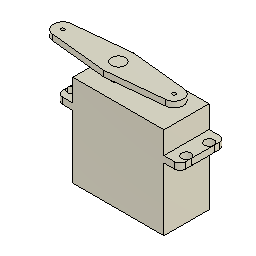
Trunk v2 (Autodesk Fusion 360 archive; units mm, degrees)
design "Servo"
Autodesk Fusion 360 part; units mm, degrees
sketch "Sketch1" plane through (0, 0, 0) normal (0, 1, 0) x (1, 0, 0)
  line L0 (0, 0) -> (39.6, 0)
  line L1 (39.6, 0) -> (39.6, -19.6)
  line L2 (39.6, -19.6) -> (0, -19.6)
  line L3 (0, -19.6) -> (0, 0)
  dimension "d1" = 19.6
  dimension "d2" = 39.6
  constraint horizontal L0
  constraint vertical L1
  constraint horizontal L2
  constraint vertical L3
  constraint coincident L0.start L3.end
  measures "d1" distance of L0.start L2.end
  measures "d2" distance of L1.end L2.end
extrude "Extrude1" add sketch "Sketch1" along normal blind 39.9 makes body 1
ref_plane "WorkPlane1" through (19.8, 27.4, 9.8) normal (0, -1, 0) x (-1, 0, 0)
sketch "Sketch2" plane through (0, 27.4, 0) normal (0, -1, 0) x (-1, 0, 0)
  line L0 (-46.6, -19.6) -> (7, -19.6)
  line L1 (7, -19.6) -> (7, 0)
  line L2 (7, 0) -> (-46.6, 0)
  line L3 (-46.6, 0) -> (-46.6, -19.6)
  line L4 (-46.6, -19.6) -> (7, 0) construction
  line L5 (7, -19.6) -> (-46.6, 0) construction
  line L6 (-19.8, -19.6) -> (-19.8, 0) construction
  line L7 (-39.6, -19.6) -> (0, -19.6) construction
  line L8 (0, 0) -> (-39.6, 0) construction
  circle A0 centre (-44.55, -14.8) radius 2.05
  circle A1 centre (-44.55, -4.8) radius 2.05
  circle A2 centre (4.95, -14.8) radius 2.05
  circle A3 centre (4.95, -4.8) radius 2.05
  line L9 (-44.55, -14.8) -> (4.95, -14.8) construction
  line L10 (4.95, -14.8) -> (4.95, -4.8) construction
  line L11 (4.95, -4.8) -> (-44.55, -4.8) construction
  line L12 (-44.55, -4.8) -> (-44.55, -14.8) construction
  line L13 (7, -9.8) -> (4.95, -9.8) construction
  point P0 (-19.8, -9.8)
  point P1 (-19.8, -14.8)
  dimension "d7" = 53.6
  dimension "d8" = 4.1
  dimension "d9" = 49.5
  dimension "d10" = 10
  constraint horizontal L0
  constraint perpendicular L0 L1
  constraint parallel L0 L2
  constraint parallel L1 L3
  constraint coincident L4 P0
  constraint coincident L5 P0
  constraint vertical L6
  constraint midpoint L6.start L7
  constraint midpoint L6.end L8
  constraint midpoint P0 L6
  constraint collinear L0 L7
  constraint horizontal L9
  constraint vertical L10
  constraint horizontal L11
  constraint vertical L12
  constraint coincident A3.centre L10.end
  constraint coincident A0.centre L9.start
  constraint coincident A1.centre L11.end
  constraint coincident A2.centre L9.end
  constraint equal A0 A1
  constraint equal A1 A3
  constraint equal A2 A3
  constraint coincident L6 P1
  constraint midpoint L9 P1
  constraint midpoint L1 L13.start
  constraint midpoint L10 L13.end
  constraint horizontal L13
  measures "d7" distance of L1 L3
  measures "d8" diameter of A0
  measures "d9" distance of A0.centre A2.centre
  measures "d10" distance of A0.centre A1.centre
extrude "Extrude2" add sketch "Sketch2" against normal blind 2.8 bodies 1
sketch "Sketch3" plane through (0, 39.9, 0) normal (0, 1, 0) x (-1, 0, 0)
  line L0 (0, 19.6) -> (-39.6, 19.6)
  line L1 (-39.6, 19.6) -> (-39.6, 0)
  line L2 (-39.6, 0) -> (0, 0)
  line L3 (0, 0) -> (0, 19.6)
  line L4 (0, 9.8) -> (-10, 9.8) construction
  circle A0 centre (-10, 9.8) radius 3
  dimension "d13" = 6
  dimension "d14" = 10
  constraint midpoint L3 L4.start
  constraint perpendicular L3 L4
  constraint coincident L4.end A0.centre
  measures "d13" diameter of A0
  measures "d14" distance of L4.start L4.end
extrude "Extrude3" add sketch "Sketch3" along normal blind 6 contours A0 bodies 1
fillet "Fillet1" radius 2.5 4 edges at (-7, 28.8, 19.6) (-7, 28.8, 0) (46.6, 28.8, 19.6) (46.6, 28.8, 0) on bodies 1
sketch "Sketch5" plane through (0, 45.9, 0) normal (0, 1, 0) x (-1, 0, 0)
  circle A0 centre (-10, 9.8) radius 3
  line L0 (6.25, 9.8) -> (-10, -6.45) construction
  line L1 (-10, -6.45) -> (-26.25, 9.8) construction
  line L2 (-26.25, 9.8) -> (-10, 26.05) construction
  line L3 (-10, 26.05) -> (6.25, 9.8) construction
  line L4 (-18.125, 17.925) -> (-1.875, 1.675) construction
  line L5 (-1.875, 17.925) -> (-18.125, 1.675) construction
  line L6 (-10, 9.8) -> (-7, 9.8) construction
  circle A1 centre (6.25, 9.8) radius 0.75
  circle A2 centre (-26.25, 9.8) radius 0.75
  circle A3 centre (-10, -6.45) radius 0.75
  circle A4 centre (-10, 26.05) radius 0.75
  line L7 (6.25, 13.8) -> (-26.25, 13.8)
  arc A5 (-26.25, 13.8) -> (-26.25, 5.8) centre (-26.25, 9.8) ccw
  line L8 (-26.25, 5.8) -> (6.25, 5.8)
  arc A6 (6.25, 5.8) -> (6.25, 13.8) centre (6.25, 9.8) ccw
  line L9 (6.25, 9.8) -> (-26.25, 9.8) construction
  line L10 (-6, -6.45) -> (-6, 26.05)
  arc A7 (-6, 26.05) -> (-14, 26.05) centre (-10, 26.05) ccw
  line L11 (-14, 26.05) -> (-14, -6.45)
  arc A8 (-14, -6.45) -> (-6, -6.45) centre (-10, -6.45) ccw
  line L12 (-10, -6.45) -> (-10, 26.05) construction
  point P0 (-10, 9.8)
  dimension "d34" = 45
  dimension "d35" = 32.5
  dimension "d36" = 1.5
  dimension "d37" = 4
  constraint perpendicular L0 L1
  constraint parallel L0 L2
  constraint parallel L1 L3
  constraint midpoint L2 L4.start
  constraint midpoint L0 L4.end
  constraint perpendicular L0 L4
  constraint midpoint L3 L5.start
  constraint midpoint L1 L5.end
  constraint coincident L4 P0
  constraint midpoint L5 P0
  constraint equal L4 L5
  constraint coincident P0 A0.centre
  constraint coincident A0 L6.end
  constraint horizontal L6
  constraint coincident L0.start L3.end
  constraint coincident L1.end L2.start
  constraint coincident L0.end L1.start
  constraint coincident L2.end L3.start
  constraint equal A2 A3
  constraint equal A1 A3
  constraint equal A1 A4
  constraint tangent L7 A5
  constraint tangent A5 L8
  constraint parallel L7 L8
  constraint tangent L8 A6
  constraint tangent L7 A6
  constraint horizontal L9
  constraint tangent L10 A7
  constraint tangent A7 L11
  constraint parallel L10 L11
  constraint tangent L11 A8
  constraint tangent L10 A8
  constraint vertical L12
  constraint equal A5 A8
  measures "d34" angle of L4 L6
  measures "d35" distance of L0.start L1.end
  measures "d36" diameter of A2
  measures "d37" radius of A8
extrude "Extrude6" add sketch "Sketch5" against normal blind 2.5 separate body makes body 2
copy_body "Body->Comp1" bodies 2 removing the originals makes body 3 in component "4 arm "
copy_body "Body->Comp2" bodies 1 removing the originals makes body 4 in component "Servo"
sketch "Sketch6" plane through (0, 45.9, 0) normal (0, 1, 0) x (-1, 0, 0)
  circle A0 centre (-10, 9.8) radius 3
  arc A1 (14.6568, 5.8207) -> (14.6568, 13.7793) centre (14.25, 9.8) ccw
  arc A2 (-34.6568, 13.7793) -> (-34.6568, 5.8207) centre (-34.25, 9.8) ccw
  line L0 (-34.25, 9.8) -> (14.25, 9.8) construction
  circle A3 centre (14.25, 9.8) radius 0.75
  circle A4 centre (-34.25, 9.8) radius 0.75
  line L1 (14.6568, 5.8207) -> (-10, 3.3)
  line L2 (-10, 3.3) -> (-34.6568, 5.8207)
  line L3 (-34.6568, 13.7793) -> (-10, 16.3)
  line L4 (-10, 16.3) -> (14.6568, 13.7793)
  line L5 (-10, 3.3) -> (-10, 16.3) construction
  circle A5 centre (-10, 9.8) radius 3
  point P0 (-10, 9.8)
  dimension "d46" = 48.5
  dimension "d48" = 1.5
  dimension "d49" = 13
  dimension "d50" = 4
  dimension "d51" = 6
  constraint horizontal L0
  constraint coincident P0 A0.centre
  constraint midpoint L0 P0
  constraint concentric A1 A3
  constraint concentric A2 A4
  constraint equal A3 A4
  constraint equal A1 A2
  constraint vertical L5
  constraint equal L1 L2
  constraint equal L3 L4
  constraint tangent A1 L1
  constraint tangent A1 L4
  constraint tangent A2 L3
  constraint midpoint P0 L5
  constraint concentric A0 A5
  measures "d46" distance of A2.centre A1.centre
  measures "d48" diameter of A3
  measures "d49" distance of L1.end L3.end
  measures "d50" radius of A1
  measures "d51" diameter of A5
extrude "Extrude7" add sketch "Sketch6" against normal blind 2.5 separate body makes body 5
copy_body "Body->Comp3" bodies 5 removing the originals makes body 6 in component "2 arm "
move_body "Move1" bodies 4 to x (1, 0, 0) y (0, 0, 1) z (0, -1, 0) at (0, 49.7, -30.1) in component "Servo"
move_body "Move1'" bodies 6 to x (1, 0, 0) y (0, 0, 1) z (0, -1, 0) at (0, 49.7, -30.1) in component "2 arm "
move_body "Move2" bodies 4 to x (1, 0, 0) y (0, 1, 0) z (0, 0, 1) at (0, -49.7, 30.1) in component "Servo"
move_body "Move2'" bodies 6 to x (1, 0, 0) y (0, 1, 0) z (0, 0, 1) at (0, -49.7, 30.1) in component "2 arm "
component "4 arm " placed x (1, 0, 0) y (0, 0, -1) z (0, 1, 0) at (0, -19.6, 89.3)
component "Servo" placed x (1, 0, 0) y (0, 1, 0) z (0, 0, 1) at (0, 0, 0)
component "2 arm " placed x (1, 0, 0) y (0, 1, 0) z (0, 0, 1) at (0, 0, 0)
equation "d19 = ( 16 * 4 ) * 1 mm"
named bodies: "Servo", "2 arm"
